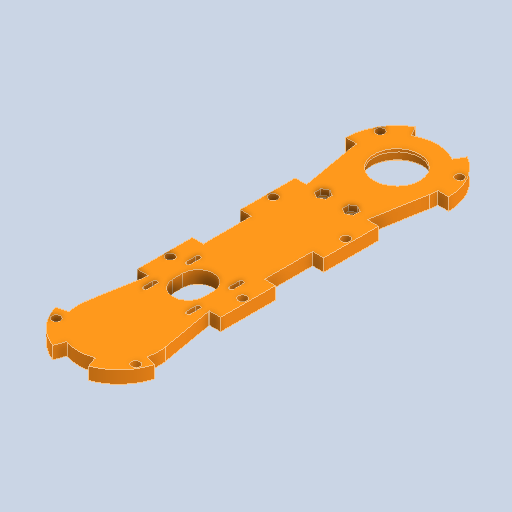
# Autodesk Inventor part: Tercer Segmento - inferior
Saved by Autodesk Inventor 2026 (Build 300175050, 175E)
## iProperties
Created: 2025-08-11
Part Number: Tercer Segmento - inferior
Material: Plastico PETG
Document SubType Name: Modeling
Designer: bello
Density: 1.27 g/cm^3
Appearance: Naranja
Author: bello
Autodesk Inventor part; units mm, degrees
ref_plane "YZ Plane" through (0, 0, 0) normal (1, 0, 0) x (0, 1, 0)
ref_plane "XZ Plane" through (0, 0, 0) normal (0, 1, 0) x (-1, 0, 0)
ref_plane "XY Plane" through (0, 0, 0) normal (0, 0, 1) x (1, 0, 0)
sketch "Boceto7" plane through (0, 0, 0) normal (0, 1, 0) x (-1, 0, 0)
  circle A0 centre (0, 0) radius 37
  circle A1 centre (0, -200) radius 37
  line L0 (0, 0) -> (0, -200)
  line L1 (0, -100) -> (11.2755, -100)
  line L2 (30, -21.6564) -> (30, -178.3436)
  line L3 (-30, -21.6564) -> (-30, -178.3436)
  line L4 (36.4379, -6.425) -> (30, -42.9361)
  line L5 (36.4379, -193.575) -> (30, -157.0639)
  line L6 (-36.4379, -6.425) -> (-30, -42.9361)
  line L7 (-36.4379, -193.575) -> (-30, -157.0639)
  dimension "d47" = 74
  dimension "d48" = 74
  dimension "d49" = 200
  dimension "d50" = 60
  dimension "d51" = 170
  constraints: 16 end point, 6 symmetric about line, 5 point on circle, 2 centre point, 2 parallel, 1 coincident, 1 horizontal, 1 midpoint, 1 perpendicular, 1 point on line, 1 tangent, 1 vertical
  measures "d47" diameter of A0
  measures "d48" diameter of A1
  measures "d49" distance of point (0, 0) L0.end
  measures "d50" distance between parallel lines of L3 L2
  measures "d51" angle of L2 L4
extrude "Extrusión5" add sketch "Boceto7" along normal blind 9
sketch "Boceto9" plane through (0, 9, 0) normal (0, 1, 0) x (1, 0, 0)
  circle A0 centre (0, 0) radius 37
  circle A1 centre (0, 0) radius 29
  arc A2 (36.4379, 193.575) -> (-36.4379, 193.575) centre (0, 200) ccw projected
  circle A3 centre (0, 200) radius 37
  circle A4 centre (0, 200) radius 29
  line L0 (0, 200) -> (0, 0)
  line L1 (0, 200) -> (-18.5, 232.0429)
  line L2 (0, 0) -> (-12.6547, -34.7686)
  line L3 (0, 0) -> (-35.7393, -9.5763)
  line L4 (-30, 157.0639) -> (-30, 42.9361) projected
  line L5 (-30, 42.9361) -> (-22, 42.9361)
  line L6 (-22, 42.9361) -> (-22, 82.9361)
  line L7 (-22, 82.9361) -> (-30, 82.9361)
  line L8 (-30, 82.9361) -> (-30, 42.9361)
  line L9 (-30, 157.0639) -> (-22, 157.0639)
  line L10 (-22, 157.0639) -> (-22, 117.0639)
  line L11 (-22, 117.0639) -> (-30, 117.0639)
  line L12 (-30, 117.0639) -> (-30, 157.0639)
  line L13 (-22.7482, 37.9927) -> (-28.5594, 5.0358)
  line L14 (-30, 42.9361) -> (-36.4379, 6.425) projected
  line L15 (-22.7482, 37.9927) -> (-22, 42.2361)
  line L16 (-22, 42.2361) -> (-22, 42.9361)
  line L17 (-23.2977, 165.1232) -> (-28.5594, 194.9642)
  line L18 (-36.4379, 193.575) -> (-30, 157.0639) projected
  line L19 (-23.2977, 165.1232) -> (-22, 157.7639)
  line L20 (-22, 157.7639) -> (-22, 157.0639)
  line L21 (0, 200) -> (18.5, 232.0429)
  line L22 (0, 0) -> (12.6547, -34.7686)
  line L23 (0, 0) -> (35.7393, -9.5763)
  line L24 (30, 42.9361) -> (22, 42.9361)
  line L25 (22, 42.9361) -> (22, 82.9361)
  line L26 (22, 82.9361) -> (30, 82.9361)
  line L27 (30, 82.9361) -> (30, 42.9361)
  line L28 (30, 157.0639) -> (22, 157.0639)
  line L29 (22, 157.0639) -> (22, 117.0639)
  line L30 (22, 117.0639) -> (30, 117.0639)
  line L31 (30, 117.0639) -> (30, 157.0639)
  line L32 (22.7482, 37.9927) -> (28.5594, 5.0358)
  line L33 (22.7482, 37.9927) -> (22, 42.2361)
  line L34 (22, 42.2361) -> (22, 42.9361)
  line L35 (23.2977, 165.1232) -> (28.5594, 194.9642)
  line L36 (23.2977, 165.1232) -> (22, 157.7639)
  line L37 (22, 157.7639) -> (22, 157.0639)
  line L38 (-22, 82.9361) -> (-22, 117.0639)
  line L39 (22, 82.9361) -> (22, 117.0639)
  line L40 (-37, 200) -> (37, 200)
  line L41 (36.4379, 6.425) -> (30, 42.9361) projected
  line L42 (30, 42.9361) -> (36.4379, 6.425)
  line L43 (30, 157.0639) -> (36.4379, 193.575) projected
  line L44 (30, 157.0639) -> (36.4379, 193.575)
  line L45 (30, 82.9361) -> (30, 117.0639)
  line L46 (30, 42.9361) -> (30, 157.0639) projected
  point P0 (14.5, 225.1147)
  point P1 (-14.5, 225.1147)
  point P2 (29, 200)
  point P3 (-29, 200)
  point P4 (28.0118, -7.5058)
  point P5 (-28.0118, -7.5058)
  point P6 (9.9186, -27.2511)
  point P7 (-9.9186, -27.2511)
  dimension "d54" = 58
  dimension "d55" = 58
  dimension "d56" = 30
  dimension "d57" = 20
  dimension "d58" = 55
  dimension "d59" = 40
  dimension "d60" = 40
  dimension "d61" = 8
  constraints: 82 end point, 17 symmetric about line, 7 parallel, 6 point on line, 5 collinear, 5 point on circle, 4 coincident, 3 perpendicular, 2 centre point, 2 horizontal, 2 tangent, 2 vertical, 8 other
  measures "d56" angle of L0 L1
  measures "d57" angle of L0 L2
  measures "d58" angle of L2 L3
  measures "d59" distance of L5.end L6.end
  measures "d60" distance of L9.end L10.end
  measures "d61" distance of L6.end L7.end
extrude "Extrusión6" cut sketch "Boceto9" against normal through all contours A0 L23 A1 L32 | A0 L32 L33 L34 L24 L41 | A0 L2 A1 L22 | L26 L39 L30 L45 | L13 A1 L3 A0 | A0 L14 L5 L16 L15 L13 | L17 L19 L20 L9 L18 A3 | A3 A2 L40 A4 L17 | L35 A4 L40 A2 A3 | A3 L43 L28 L37 L36 L35 | L4 L11 L38 L7 | L1 A2 L21 A4
sketch "Boceto10" plane through (0, 9, 0) normal (0, 1, 0) x (1, 0, 0)
  circle A0 centre (0, 0) radius 33
  arc A1 (14.5, 225.1147) -> (-14.5, 225.1147) centre (0, 200) ccw projected
  circle A2 centre (0, 200) radius 33
  circle A3 centre (-28.5788, 216.5) radius 2.05
  circle A4 centre (-26, 137.0639) radius 2.05
  circle A5 centre (-26, 62.9361) radius 2.05
  circle A6 centre (-28.5788, -16.5) radius 2.05
  line L0 (0, 0) -> (0, 200)
  line L1 (-22, 82.9361) -> (-30, 82.9361) projected
  line L2 (-30, 82.9361) -> (-30, 42.9361) projected
  line L3 (-30, 117.0639) -> (-22, 117.0639) projected
  line L4 (-30, 157.0639) -> (-30, 117.0639) projected
  line L5 (0, 200) -> (-28.5788, 216.5)
  line L6 (0, 0) -> (-28.5788, -16.5)
  circle A7 centre (28.5788, 216.5) radius 2.05
  circle A8 centre (26, 137.0639) radius 2.05
  circle A9 centre (26, 62.9361) radius 2.05
  circle A10 centre (28.5788, -16.5) radius 2.05
  circle A11 centre (0, 200) radius 16.5
  dimension "d64" = 66
  dimension "d65" = 66
  dimension "d66" = 4.1
  dimension "d67" = 20
  dimension "d68" = 4
  dimension "d69" = 20
  dimension "d70" = 4
  dimension "d71" = 60
  dimension "d72" = 60
  dimension "d73" = 33
  constraints: 9 centre point, 6 end point, 4 symmetric about line, 3 coincident, 3 equal radius, 1 vertical, 10 other
  measures "d66" diameter of A5
  measures "d67" distance from line of L1 A5.centre
  measures "d68" distance from line of L2 A5.centre
  measures "d69" distance from line of L3 A4.centre
  measures "d70" distance from line of L4 A4.centre
  measures "d71" angle of L5 L0
  measures "d72" angle of L0 L6
  measures "d73" diameter of A11
extrude "Extrusión7" cut sketch "Boceto10" against normal through all contours A10 A0 | A0 A10 | A6 L6 A0 | A0 A6 | L6 A6 A0 | A7 A2 | A2 A7 | A3 A2 | A2 L5 A3 | A11 L5 L0 | L0 L5 A11 | A3 L5 A2 | A4 | A5 | A8 | A9
sketch "Boceto11" plane through (0, 9, 0) normal (0, 1, 0) x (1, 0, 0)
  circle A0 centre (-28.5788, -16.5) radius 2.05 projected
  circle A1 centre (-28.5788, -16.5) radius 3.1
  circle A2 centre (28.5788, -16.5) radius 2.05 projected
  circle A3 centre (28.5788, -16.5) radius 3.1
  circle A4 centre (26, 62.9361) radius 2.05 projected
  circle A5 centre (26, 62.9361) radius 3.1
  circle A6 centre (-26, 62.9361) radius 2.05 projected
  circle A7 centre (-26, 62.9361) radius 3.1
  circle A8 centre (-26, 137.0639) radius 2.05 projected
  circle A9 centre (-26, 137.0639) radius 3.1
  circle A10 centre (26, 137.0639) radius 2.05 projected
  circle A11 centre (26, 137.0639) radius 3.1
  circle A12 centre (28.5788, 216.5) radius 2.05 projected
  circle A13 centre (28.5788, 216.5) radius 3.1
  circle A14 centre (-28.5788, 216.5) radius 2.05 projected
  circle A15 centre (-28.5788, 216.5) radius 3.1
  point P0 (0, 0)
  dimension "d76" = 6.2
  dimension "d77" = 6.2
  dimension "d78" = 6.2
  dimension "d79" = 6.2
  dimension "d80" = 6.2
  dimension "d81" = 6.2
  dimension "d82" = 6.2
  dimension "d83" = 6.2
  constraints: 8 centre point, 8 coincident
  measures "d76" diameter of A1
  measures "d77" diameter of A3
  measures "d78" diameter of A5
  measures "d79" diameter of A7
  measures "d80" diameter of A9
  measures "d81" diameter of A11
  measures "d82" diameter of A13
  measures "d83" diameter of A15
extrude "Extrusión8" cut sketch "Boceto11" against normal blind 5 contours A0 | A1 | A2 | A3 | A4 | A5 | A6 | A7 | A8 | A9 | A10 | A11 | A12 | A13 | A14 | A15
sketch "Boceto12" plane through (0, 9, 0) normal (0, 1, 0) x (1, 0, 0)
  line L0 (11.1, 50) -> (11.1, 57)
  line L1 (-11.1, 57) -> (-11.1, 50)
  arc A0 (-11.1, 50) -> (11.1, 50) centre (0, 50) ccw
  arc A1 (11.1, 57) -> (-11.1, 57) centre (0, 57) ccw
  line L2 (-15.5, 41.5) -> (-15.5, 34.5) construction
  line L3 (-17.05, 41.5) -> (-17.05, 34.5)
  line L4 (-13.95, 34.5) -> (-13.95, 41.5)
  arc A2 (-13.95, 41.5) -> (-17.05, 41.5) centre (-15.5, 41.5) ccw
  arc A3 (-17.05, 34.5) -> (-13.95, 34.5) centre (-15.5, 34.5) ccw
  circle A4 centre (0, 200) radius 16.5 projected
  line L5 (0, 200) -> (-8.0711, 200)
  line L6 (0, 50) -> (-7.1529, 50)
  line L7 (0, 50) -> (0, 43.05)
  line L8 (15.5, 41.5) -> (15.5, 34.5) construction
  line L9 (17.05, 41.5) -> (17.05, 34.5)
  line L10 (13.95, 34.5) -> (13.95, 41.5)
  arc A5 (17.05, 41.5) -> (13.95, 41.5) centre (15.5, 41.5) ccw
  arc A6 (13.95, 34.5) -> (17.05, 34.5) centre (15.5, 34.5) ccw
  line L11 (0, 50) -> (0, 57)
  line L12 (0, 53.5) -> (-7.1529, 53.5)
  line L13 (-15.5, 65.5) -> (-15.5, 72.5) construction
  line L14 (-17.05, 65.5) -> (-17.05, 72.5)
  line L15 (-13.95, 72.5) -> (-13.95, 65.5)
  arc A7 (-17.05, 65.5) -> (-13.95, 65.5) centre (-15.5, 65.5) ccw
  arc A8 (-13.95, 72.5) -> (-17.05, 72.5) centre (-15.5, 72.5) ccw
  arc A9 (13.95, 65.5) -> (17.05, 65.5) centre (15.5, 65.5) ccw
  line L16 (15.5, 65.5) -> (15.5, 72.5) construction
  line L17 (13.95, 72.5) -> (13.95, 65.5)
  line L18 (17.05, 65.5) -> (17.05, 72.5)
  arc A10 (17.05, 72.5) -> (13.95, 72.5) centre (15.5, 72.5) ccw
  point P0 (0, 0)
  point P1 (-15.5, 38)
  point P2 (15.5, 38)
  point P3 (-15.5, 69)
  point P4 (15.5, 69)
  dimension "d86" = 7
  dimension "d87" = 22.2
  dimension "d89" = 7
  dimension "d90" = 3.1
  dimension "d128" = 12
  dimension "d129" = 15.5
  dimension "d130" = 150
  constraints: 46 end point, 21 symmetric about line, 20 point on circle, 10 centre point, 8 tangent, 3 horizontal, 3 parallel, 2 midpoint, 2 vertical, 6 other
  measures "d86" distance of L1.start L1.end
  measures "d87" distance between parallel lines of L0 L1
  measures "d89" distance of L3.start L3.end
  measures "d90" distance between parallel lines of L4 L3
  measures "d128" distance from line of point (-15.5, 38) L6
  measures "d129" distance from line of L7 point (-15.5, 38)
  measures "d130" distance of L5.start L6.start
extrude "Extrusión9" cut sketch "Boceto12" against normal through all contours A0 L1 A1 L0 | A2 L4 A3 L3 | L9 A6 L10 A5 | L14 A8 L15 A7 | L17 A10 L18 A9
sketch "Boceto13" plane through (0, 9, 0) normal (0, 1, 0) x (1, 0, 0)
  line L0 (-22, 157.7639) -> (-22, 157.0639) projected
  line L1 (30, 157.0639) -> (22, 157.0639) projected
  line L2 (-22, 157.0639) -> (22, 157.0639)
  circle A0 centre (0, 200) radius 16.5 projected
  circle A1 centre (0, 200) radius 25.5
  circle A2 centre (-10, 157.0639) radius 2.6
  circle A3 centre (10, 157.0639) radius 2.6
  line L3 (30, 117.0639) -> (30, 157.0639) projected
  line L4 (-30, 157.0639) -> (-30, 117.0639) projected
  line L5 (-11.1, 50) -> (-11.1, 57) projected
  line L6 (-7.4, 157.0639) -> (-22.9107, 188.804)
  line L7 (7.4, 157.0639) -> (22.9107, 188.804)
  arc A4 (11.1, 57) -> (-11.1, 57) centre (0, 57) ccw projected
  line L8 (-11.1, 57) -> (11.1, 57)
  circle A5 centre (0, 57) radius 5
  line L9 (-7.4, 157.0639) -> (-5, 57)
  line L10 (7.4, 157.0639) -> (5, 57)
  point P0 (0, 0)
  point P1 (-11.1, 53.5)
  point P2 (0, 57)
  dimension "d96" = 5.2
  dimension "d95" = 51
  dimension "d97" = 20
  dimension "d98" = 20
  dimension "d100" = 35.3272
  dimension "d102" = 10
  dimension "d103" = 143
  dimension "d104" = 100.0927
  constraints: 12 end point, 6 point on line, 4 point on circle, 2 centre point, 2 coincident, 2 horizontal, 2 horizontal alignment, 2 midpoint, 2 tangent, 4 other
  measures "d95" diameter of A1
  measures "d97" distance from line of L3 point (10, 157.064)
  measures "d98" distance from line of L4 point (-10, 157.064)
  measures "d100" distance of L6.start L6.end
  measures "d102" diameter of A5
  measures "d103" distance of point (0, 57) A1.centre
  measures "d104" distance of L6.start L9.end
extrude "Extrusión10" cut sketch "Boceto13" against normal blind 10 contours A2 L2 | L6 A2 | L2 A2 L6 | L7 A3 L2 | L2 A3 | A3 L7
sketch "Boceto16" plane through (0, 0, 0) normal (0, -1, 0) x (1, 0, 0)
  circle A0 centre (0, -200) radius 16.5 projected
  circle A1 centre (0, -200) radius 18.5
  point P0 (0, 0)
  dimension "d108" = 37
  constraints: 1 centre point, 1 coincident
  measures "d108" diameter of A1
extrude "Extrusión11" cut sketch "Boceto16" against normal blind 7
sketch "Boceto17" plane through (0, 9, 0) normal (0, 1, 0) x (1, 0, 0)
  line L0 (-30, 82.9361) -> (-22, 82.9361) projected
  line L1 (-30, 82.9361) -> (-22, 82.9361)
  line L2 (-22, 82.9361) -> (-22, 82.6861)
  line L3 (-22, 82.6861) -> (-30, 82.6861)
  line L4 (-30, 82.6861) -> (-30, 82.9361)
  line L5 (-22, 42.9361) -> (-30, 42.9361) projected
  line L6 (-30, 42.9361) -> (-22, 42.9361)
  line L7 (-22, 42.9361) -> (-22, 43.1861)
  line L8 (-22, 43.1861) -> (-30, 43.1861)
  line L9 (-30, 43.1861) -> (-30, 42.9361)
  line L10 (-22, 117.0639) -> (-30, 117.0639) projected
  line L11 (-30, 117.0639) -> (-22, 117.0639)
  line L12 (-22, 117.0639) -> (-22, 117.3139)
  line L13 (-22, 117.3139) -> (-30, 117.3139)
  line L14 (-30, 117.3139) -> (-30, 117.0639)
  line L15 (-30, 157.0639) -> (-30, 117.0639) projected
  line L16 (-30, 157.0639) -> (-22, 157.0639)
  line L17 (-22, 157.0639) -> (-22, 156.8139)
  line L18 (-22, 156.8139) -> (-30, 156.8139)
  line L19 (-30, 156.8139) -> (-30, 157.0639)
  line L20 (-29, 200) -> (-37, 200) projected
  line L21 (-37, 200) -> (-29, 200)
  line L22 (-29, 200) -> (-29, 200.25)
  line L23 (-29, 200.25) -> (-37, 200.25)
  line L24 (-37, 200.25) -> (-37, 200)
  line L25 (-35.7393, -9.5763) -> (-28.0118, -7.5058) projected
  line L26 (-28.0118, -7.5058) -> (-27.9471, -7.7472)
  line L27 (-27.9471, -7.7472) -> (-35.6746, -9.8178)
  line L28 (-35.7393, -9.5763) -> (-35.6746, -9.8178)
  line L29 (-9.9186, -27.2511) -> (-10.1535, -27.1656)
  line L30 (-12.6547, -34.7686) -> (-9.9186, -27.2511) projected
  line L31 (-10.1535, -27.1656) -> (-12.8897, -34.6831)
  arc A0 (-35.7393, -9.5763) -> (-12.6547, -34.7686) centre (0, 0) ccw projected
  line L32 (-12.6547, -34.7686) -> (-12.8897, -34.6831)
  line L33 (-18.5, 232.0429) -> (-14.5, 225.1147) projected
  line L34 (-14.5, 225.1147) -> (-14.7165, 224.9897)
  line L35 (-14.7165, 224.9897) -> (-18.7165, 231.9179)
  line L36 (-18.5, 232.0429) -> (-18.7165, 231.9179)
  line L37 (0, 0) -> (0, 200)
  line L38 (30, 82.9361) -> (22, 82.9361)
  line L39 (30, 82.9361) -> (22, 82.9361)
  line L40 (22, 82.9361) -> (22, 82.6861)
  line L41 (22, 82.6861) -> (30, 82.6861)
  line L42 (30, 82.6861) -> (30, 82.9361)
  line L43 (22, 42.9361) -> (30, 42.9361)
  line L44 (30, 42.9361) -> (22, 42.9361)
  line L45 (22, 42.9361) -> (22, 43.1861)
  line L46 (22, 43.1861) -> (30, 43.1861)
  line L47 (30, 43.1861) -> (30, 42.9361)
  line L48 (22, 117.0639) -> (30, 117.0639)
  line L49 (30, 117.0639) -> (22, 117.0639)
  line L50 (22, 117.0639) -> (22, 117.3139)
  line L51 (22, 117.3139) -> (30, 117.3139)
  line L52 (30, 117.3139) -> (30, 117.0639)
  line L53 (30, 157.0639) -> (30, 117.0639)
  line L54 (30, 157.0639) -> (22, 157.0639)
  line L55 (22, 157.0639) -> (22, 156.8139)
  line L56 (22, 156.8139) -> (30, 156.8139)
  line L57 (30, 156.8139) -> (30, 157.0639)
  line L58 (29, 200) -> (37, 200)
  line L59 (37, 200) -> (29, 200)
  line L60 (29, 200) -> (29, 200.25)
  line L61 (29, 200.25) -> (37, 200.25)
  line L62 (37, 200.25) -> (37, 200)
  line L63 (35.7393, -9.5763) -> (28.0118, -7.5058)
  line L64 (28.0118, -7.5058) -> (27.9471, -7.7472)
  line L65 (27.9471, -7.7472) -> (35.6746, -9.8178)
  line L66 (35.7393, -9.5763) -> (35.6746, -9.8178)
  line L67 (9.9186, -27.2511) -> (10.1535, -27.1656)
  line L68 (12.6547, -34.7686) -> (9.9186, -27.2511)
  line L69 (10.1535, -27.1656) -> (12.8897, -34.6831)
  line L70 (12.6547, -34.7686) -> (12.8897, -34.6831)
  line L71 (18.5, 232.0429) -> (14.5, 225.1147)
  line L72 (14.5, 225.1147) -> (14.7165, 224.9897)
  line L73 (14.7165, 224.9897) -> (18.7165, 231.9179)
  line L74 (18.5, 232.0429) -> (18.7165, 231.9179)
  point P0 (-12.8894, -34.6823)
  dimension "d111" = 0.25
  constraints: 134 end point, 36 symmetric about line, 14 perpendicular, 10 parallel, 7 equal length, 6 point on line, 5 horizontal, 1 tangent, 1 vertical
  measures "d111" distance of L16.end L17.end
extrude "Extrusión12" cut sketch "Boceto17" against normal through all
chamfer "Chaflán1" distance 0.7 angle 45 1 edges at (-18.5, 0, -200)
sketch "Boceto19" plane through (0, 9, 0) normal (0, 1, 0) x (1, 0, 0)
  circle A0 centre (-10, 157.0639) radius 2.6 projected
  line L0 (-10, 161.7405) -> (-5.95, 159.4022)
  line L1 (-5.95, 159.4022) -> (-5.95, 154.7257)
  line L2 (-5.95, 154.7257) -> (-10, 152.3874)
  line L3 (-10, 152.3874) -> (-14.05, 154.7257)
  line L4 (-14.05, 154.7257) -> (-14.05, 159.4022)
  line L5 (-14.05, 159.4022) -> (-10, 161.7405)
  circle A1 centre (10, 157.0639) radius 2.6 projected
  line L6 (10, 161.7405) -> (14.05, 159.4022)
  line L7 (14.05, 159.4022) -> (14.05, 154.7257)
  line L8 (14.05, 154.7257) -> (10, 152.3874)
  line L9 (10, 152.3874) -> (5.95, 154.7257)
  line L10 (5.95, 154.7257) -> (5.95, 159.4022)
  line L11 (5.95, 159.4022) -> (10, 161.7405)
  point P0 (0, 0)
  dimension "d121" = 8.1
  constraints: 24 end point, 2 coincident, 1 parallel, 26 other
  measures "d121" distance between parallel lines of L1 L4
extrude "Extrusión14" cut sketch "Boceto19" against normal blind 4 contours A0 | L0 L1 L2 L3 L4 L5 | A1 | L6 L7 L8 L9 L10 L11
